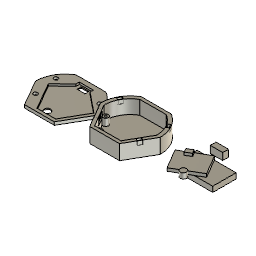
LampPost_Enclosure v37 (Autodesk Fusion 360 design; units mm, degrees)
Autodesk Fusion 360 part; units mm, degrees
note: some values were not read from the file. Set by a fixed rule: which sketch regions a step uses.
sketch "Sketch1" plane through (0, 0, 0) normal (0, 0, 1) x (1, 0, 0)
  line L0 (17.2286, 28.7143) -> (-16.253, 29.2775)
  line L1 (-33.4816, 0.5632) -> (-17.2286, -28.7143)
  line L2 (-17.2286, -28.7143) -> (16.253, -29.2775)
  line L3 (16.253, -29.2775) -> (33.4816, -0.5632)
  line L4 (19.6049, 32.6749) -> (-18.4948, 33.3158)
  line L5 (-38.0997, 0.6409) -> (-19.6049, -32.6749)
  line L6 (-19.6049, -32.6749) -> (18.4948, -33.3158)
  line L7 (18.4948, -33.3158) -> (38.0997, -0.6409)
  circle A0 centre (0, 0) radius 33.4863
  circle A1 centre (0, 0) radius 38.1051
  dimension "d1" = 29
  dimension "d2" = 33
  constraint coincident A0.centre A1.centre
  constraint coincident L3.end A0
  constraint coincident L7.end A1
  measures "d1" distance of A0.centre L3
  measures "d2" distance of A0.centre L7
extrude "Extrude1" add sketch "Sketch1" along normal blind 19 contours L0 L1 L2 L3 A0 | L4 L7 A0 A1 | L0 L4 A0 | L4 L5 A0 A1 | L1 L5 A0 | L3 L7 A0 | L5 L6 A0 | L2 L6 A0 | L6 L7 A0 makes body 1
sketch "Sketch2" plane through (0, 0, 19) normal (0, 0, 1) x (-1, 0, 0)
  arc A0 (-38.0997, 0.6409) -> (-19.6049, -32.6749) centre (0, 0) ccw
  line L0 (-19.6049, -32.6749) -> (18.4948, -33.3158)
  arc A1 (18.4948, -33.3158) -> (38.0997, -0.6409) centre (0, 0) ccw
  line L1 (38.0997, -0.6409) -> (19.6049, 32.6749)
  line L2 (19.6049, 32.6749) -> (-18.4948, 33.3158)
  line L3 (-18.4948, 33.3158) -> (-38.0997, 0.6409)
  line L4 (17.1219, 28.778) -> (-16.3615, 29.217)
  line L5 (-16.3615, 29.217) -> (-33.4834, 0.439)
  line L6 (-33.4834, 0.439) -> (-17.1219, -28.778)
  line L7 (-17.1219, -28.778) -> (16.3615, -29.217)
  line L8 (16.3615, -29.217) -> (33.4834, -0.439)
  line L9 (33.4834, -0.439) -> (17.1219, 28.778)
  line L10 (19.4836, 32.7474) -> (-18.6183, 33.2469)
  line L11 (-18.6183, 33.2469) -> (-38.1018, 0.4996)
  line L12 (-19.4836, -32.7474) -> (18.6183, -33.2469)
  line L13 (38.1018, -0.4996) -> (19.4836, 32.7474)
  circle A2 centre (0, 0) radius 33.4863
  dimension "d5" = 29
  dimension "d6" = 33
  constraint coincident A0.centre A1.centre
  constraint coincident L8.end A2
  measures "d5" distance of A0.centre L9
  measures "d6" distance of A0.centre L13
extrude "Extrude2" cut sketch "Sketch2" against normal blind 17.5 contours L4 L5 L6 L7 L8 L9 | L6 A2 | L8 A2 bodies 1
sketch "Sketch3" plane through (0, 0, 1.5) normal (0, 0, 1) x (-1, 0, 0)
  line L0 (33.4834, -0.439) -> (17.1219, 28.778)
  line L1 (17.1219, 28.778) -> (-16.3615, 29.217)
  line L2 (-16.3615, 29.217) -> (-33.4834, 0.439)
  arc A0 (-33.4834, 0.439) -> (-17.1219, -28.778) centre (0, 0) ccw
  line L3 (-17.1219, -28.778) -> (16.3615, -29.217)
  arc A1 (16.3615, -29.217) -> (33.4834, -0.439) centre (0, 0) ccw
  line L4 (133, 19.0526) -> (100, 38.1051)
  line L5 (67, 19.0526) -> (67, -19.0526)
  line L6 (67, -19.0526) -> (100, -38.1051)
  line L7 (100, -38.1051) -> (133, -19.0526)
  circle A2 centre (100, 0) radius 38.1051
  point P0 (100, 0)
  constraint coincident P0 A2.centre
  constraint coincident L4.start A2
extrude "Extrude3" add sketch "Sketch3" along normal blind 4 separate body contours L4 L5 L6 L7 A2 makes body 2
sketch "Sketch4" plane through (0, 0, 19) normal (0, 0, 1) x (-1, 0, 0)
  line L0 (-16.3615, 29.217) -> (17.1219, 28.778)
  line L1 (17.1219, 28.778) -> (33.4834, -0.439)
  arc A0 (16.3615, -29.217) -> (33.4834, -0.439) centre (0, 0) ccw
  line L2 (16.3615, -29.217) -> (-17.1219, -28.778)
  arc A1 (-33.4834, 0.439) -> (-17.1219, -28.778) centre (0, 0) ccw
  line L3 (-33.4834, 0.439) -> (-16.3615, 29.217)
  arc A2 (-38.0997, 0.6409) -> (-19.6049, -32.6749) centre (0, 0) ccw
  line L4 (-19.6049, -32.6749) -> (18.4948, -33.3158)
  arc A3 (18.4948, -33.3158) -> (38.0997, -0.6409) centre (0, 0) ccw
  line L5 (38.0997, -0.6409) -> (19.6049, 32.6749)
  line L6 (19.6049, 32.6749) -> (-18.4948, 33.3158)
  line L7 (-18.4948, 33.3158) -> (-38.0997, 0.6409)
  line L8 (-17.1219, -28.778) -> (-0.3802, -28.9975) construction
  line L9 (-0.3802, -28.9975) -> (-0.5551, -32.9953) construction
  line L10 (-17.1219, -28.778) -> (-17.155, -30.7472) construction
  line L11 (-17.155, -30.7472) -> (-0.4676, -30.9964) construction
  line L12 (-16.3615, 29.217) -> (0.3802, 28.9975) construction
  line L13 (0.3802, 28.9975) -> (0.5551, 32.9953) construction
  line L14 (17.1219, 28.778) -> (17.155, 30.7467) construction
  line L15 (17.155, 30.7467) -> (0.4676, 30.9964) construction
  line L16 (17.1219, 28.778) -> (25.3026, 14.1696) construction
  line L17 (25.3026, 14.1696) -> (28.8523, 16.017) construction
  line L18 (17.1219, 28.778) -> (18.8976, 29.7638)
  line L19 (18.8976, 29.7638) -> (27.0775, 15.0933) construction
  line L20 (-33.4834, 0.439) -> (-24.9226, 14.8279) construction
  line L21 (-24.9226, 14.8279) -> (-28.2973, 16.9784) construction
  line L22 (-33.4834, 0.439) -> (-35.225, 1.4839) construction
  line L23 (-35.225, 1.4839) -> (-26.6099, 15.9031) construction
  dimension "d12" = 1.9695
  dimension "d13" = 1.969
  dimension "d14" = 16.743
  dimension "d15" = 2.031
  dimension "d16" = 16.743
  dimension "d17" = 2.031
  constraint coincident L2.end A1.end
  constraint midpoint L2 L8.end
  constraint midpoint L4 L9.end
  constraint perpendicular L4 L10
  constraint midpoint L9 L11.end
  constraint coincident L0.start L3.end
  constraint midpoint L0 L12.end
  constraint midpoint L6 L13.end
  constraint coincident L0.end L1.start
  constraint perpendicular L6 L14
  constraint midpoint L13 L15.end
  constraint parallel L1 L16
  constraint midpoint L5 L17.end
  constraint perpendicular L5 L18
  constraint midpoint L17 L19.end
  constraint coincident A1.start L3.start
  constraint parallel L3 L20
  constraint midpoint L7 L21.end
  constraint perpendicular L7 L22
  constraint midpoint L21 L23.end
  measures "d12" distance of L2.end L10.end
  measures "d13" distance of L0.end L14.end
  measures "d14" distance of L0.end L16.end
  measures "d15" distance of L0.end L18.end
  measures "d16" distance of A1.start L20.end
  measures "d17" distance of A1.start L22.end
sketch "Sketch5" plane through (0, 0, 0) normal (0, 0, 1) x (1, 0, 0)
  line L0 (130, 0) -> (100, 0)
  line L1 (100, 0) -> (100, 50)
  line L2 (100, 50) -> (130, 50)
  line L3 (130, 50) -> (130, 0)
  dimension "d18" = 30
  dimension "d19" = 50
  constraint horizontal L0
  constraint vertical L1
  constraint horizontal L2
  constraint vertical L3
  measures "d18" distance of L0.start L0.end
  measures "d19" distance of L0.start L2.end
extrude "Extrude4" add sketch "Sketch5" along normal blind 7 separate body makes body 3
move_body "Move1" bodies 3 to x (0, 1, 0) y (-1, 0, 0) z (0, 0, 1) at (24.4081, -110.5598, 0)
move_body "Move2" bodies 3 to x (1, 0, 0) y (0, 1, 0) z (0, 0, 1) at (0, 0, 1.5)
sketch "Sketch6" plane through (0, 0, 19) normal (0, 0, 1) x (-1, 0, 0)
  line L0 (-100, 0) -> (-63, 0)
  line L1 (-63, 0) -> (-63, -29)
  line L2 (-63, -29) -> (-100, -29)
  line L3 (-100, -29) -> (-100, 0)
  line L4 (-100, 0) -> (-90, 0)
  line L5 (-90, 0) -> (-82, 0)
  line L6 (-82, 0) -> (-82, -6)
  line L7 (-82, -6) -> (-90, -6)
  line L8 (-90, -6) -> (-90, 0)
  dimension "d22" = 37
  dimension "d23" = 29
  dimension "d24" = 10
  dimension "d25" = 8
  dimension "d26" = 6
  constraint horizontal L0
  constraint vertical L1
  constraint horizontal L2
  constraint vertical L3
  constraint perpendicular L3 L4
  constraint horizontal L5
  constraint vertical L6
  constraint horizontal L7
  constraint vertical L8
  measures "d22" distance of L0.start L0.end
  measures "d23" distance of L0.start L2.end
  measures "d24" distance of L0.start L4.end
  measures "d25" distance of L4.end L5.end
  measures "d26" distance of L4.end L7.end
extrude "Extrude5" add sketch "Sketch6" along normal blind 4 separate body makes body 4
sketch "Sketch7" plane through (0, 0, 23) normal (0, 0, 1) x (-1, 0, 0)
  line L0 (-63, 0) -> (-100, 0)
  line L1 (-100, 0) -> (-100, -29)
  line L2 (-100, -29) -> (-63, -29)
  line L3 (-63, -29) -> (-63, 0)
  line L4 (-90, -1) -> (-82, -1)
  line L5 (-82, -1) -> (-82, -7)
  line L6 (-82, -7) -> (-90, -7)
  line L7 (-90, -7) -> (-90, -1)
  constraint horizontal L4
  constraint vertical L5
  constraint horizontal L6
  constraint vertical L7
move_body "Move3" bodies 4 to x (1, 0, 0) y (0, 1, 0) z (0, 0, 1) at (0, 0.8273, 0)
extrude "Extrude6" add sketch "Sketch7" along normal blind 3.5 contours L4 L5 L6 L7 bodies 4
move_body "Move4" bodies 4 to x (-0.017452, -0.999848, 0) y (0.999848, -0.017452, 0) z (0, 0, 1) at (-14.8475, 71.7391, 0)
move_body "Move5" bodies 4 to x (1, 0, 0) y (0, 1, 0) z (0, 0, 1) at (0.467, -0.1168, 0)
move_body "Move6" bodies 4 to x (1, 0, 0) y (0, 1, 0) z (0, 0, 1) at (0, 0, -7.5)
move_body "Move7" bodies 4 to x (1, 0, 0) y (0, 1, 0) z (0, 0, 1) at (0, 0, -5)
move_body "Move8" bodies 4 to x (1, 0, 0) y (0, 1, 0) z (0, 0, 1) at (0, 0, 5)
move_body "Move9" bodies 4 3 to x (1, 0, 0) y (0, 1, 0) z (0, 0, 1) at (95, 0, 0)
move_body "Move10" bodies 4 to x (1, 0, 0) y (0, 1, 0) z (0, 0, 1) at (0, 0, -3)
move_body "Move11" bodies 4 to x (1, 0, 0) y (0, 1, 0) z (0, 0, 1) at (0, 0, 0.5)
move_body "Move12" bodies 4 3 to x (1, 0, 0) y (0, 1, 0) z (0, 0, 1) at (-95, 0, 0)
sketch "Sketch8" plane through (0, 0, 0) normal (0, 0, 1) x (1, 0, 0)
  line L0 (0, 70) -> (-7.5, 70)
  line L1 (-7.5, 70) -> (-7.5, 86)
  line L2 (-7.5, 86) -> (0, 86)
  line L3 (0, 86) -> (0, 70)
  dimension "d31" = 7.5
  dimension "d32" = 16
  constraint horizontal L0
  constraint vertical L1
  constraint horizontal L2
  constraint vertical L3
  measures "d31" distance of L0.start L0.end
  measures "d32" distance of L0.start L2.end
extrude "Extrude7" add sketch "Sketch8" along normal blind 9 separate body makes body 5
move_body "Move13" bodies 5 to x (0, -1, 0) y (1, 0, 0) z (0, 0, 1) at (-78.7049, 19.5356, 12.5)
sketch "Sketch9" plane through (0, 0, 0) normal (0, 0, 1) x (1, 0, 0)
  circle A0 centre (0, -50) radius 4
  dimension "d35" = 8
  measures "d35" diameter of A0
extrude "Extrude8" add sketch "Sketch9" along normal blind 7 separate body makes body 6
move_body "Move14" bodies 6 to x (1, 0, 0) y (0, 1, 0) z (0, 0, 1) at (0, 52, 14)
move_body "Move15" bodies 6 3 4 to x (1, 0, 0) y (0, 1, 0) z (0, 0, 1) at (80, 0, 0)
move_body "Move16" bodies 6 to x (1, 0, 0) y (0, 1, 0) z (0, 0, 1) at (0, 0, -1)
move_body "Move17" bodies 6 4 3 to x (1, 0, 0) y (0, 1, 0) z (0, 0, 1) at (-80, 0, 0)
move_body "Move18" bodies 4 to x (0.5, -0.866025, 0) y (0.866025, 0.5, 0) z (0, 0, 1) at (17.3641, -27.6904, 0)
move_body "Move19" bodies 4 to x (1, 0, 0) y (0, 1, 0) z (0, 0, 1) at (-17.4314, 28.0362, 0)
move_body "Move20" bodies 3 to x (1, 0, 0) y (0, 1, 0) z (0, 0, 1) at (1.0034, -1.8395, 0)
move_body "Move21" bodies 6 to x (1, 0, 0) y (0, 1, 0) z (0, 0, 1) at (-0.2172, -24.4176, 0)
move_body "Move22" bodies 6 to x (1, 0, 0) y (0, 1, 0) z (0, 0, 1) at (0, 0, -1)
move_body "Move23" bodies 6 5 4 3 to x (1, 0, 0) y (0, 1, 0) z (0, 0, 1) at (110, 0, 0)
move_body "Move24" bodies 1 to x (0.999848, 0.017452, 0) y (-0.017452, 0.999848, 0) z (0, 0, 1) at (-0.5872, 0.6599, 0)
sketch "Sketch10" plane through (0, 0, 19) normal (0, 0, 1) x (-1, 0, 0)
  line L0 (-16.2817, 28.2672) -> (17.2043, 28.4126)
  line L1 (17.2043, 28.4126) -> (34.0732, -0.5144)
  arc A0 (17.4562, -29.5869) -> (34.0732, -0.5144) centre (0.5872, -0.6599) ccw
  line L2 (17.4562, -29.5869) -> (-16.0298, -29.7323)
  arc A1 (-32.8988, -0.8053) -> (-16.0298, -29.7323) centre (0.5872, -0.6599) ccw
  line L3 (-32.8988, -0.8053) -> (-16.2817, 28.2672)
  arc A2 (-37.5179, -0.684) -> (-18.4444, -33.6719) centre (0.5872, -0.6599) ccw
  line L4 (-18.4444, -33.6719) -> (19.6607, -33.6478)
  arc A3 (19.6607, -33.6478) -> (38.6924, -0.6358) centre (0.5872, -0.6599) ccw
  line L5 (38.6924, -0.6358) -> (19.6189, 32.3522)
  line L6 (19.6189, 32.3522) -> (-18.4862, 32.3281)
  line L7 (-18.4862, 32.3281) -> (-37.5179, -0.684)
  line L8 (17.4562, -29.5869) -> (0.7133, -29.6596) construction
  line L9 (17.4562, -29.5869) -> (17.4575, -31.6179) construction
  line L10 (17.4575, -31.6179) -> (0.7132, -31.6285) construction
  line L11 (0.7132, -31.6285) -> (0.7133, -29.6596) construction
  line L12 (0.7132, -31.6285) -> (0.7142, -33.2285)
  line L13 (0.7132, -31.6285) -> (0.7122, -30.0285)
  line L14 (0.7142, -33.2285) -> (-1.8858, -33.2301)
  line L15 (0.7122, -30.0285) -> (-1.8878, -30.0301)
  line L16 (-1.8878, -30.0301) -> (-1.8858, -33.2301)
  line L17 (0.7142, -33.2285) -> (3.3142, -33.2268)
  line L18 (0.7122, -30.0285) -> (3.3122, -30.0268)
  line L19 (3.3142, -33.2268) -> (3.3122, -30.0268)
  line L20 (-16.2817, 28.2672) -> (-24.5901, 13.7311) construction
  line L21 (-24.5901, 13.7311) -> (-26.2996, 14.7082) construction
  line L22 (-26.2996, 14.7082) -> (-27.6858, 15.5073)
  line L23 (-26.2996, 14.7082) -> (-24.9105, 13.9142)
  line L24 (-27.6858, 15.5073) -> (-26.3872, 17.7598)
  line L25 (-24.9105, 13.9142) -> (-23.6203, 16.1715)
  line L26 (-27.6858, 15.5073) -> (-28.9843, 13.2548)
  line L27 (-24.9105, 13.9142) -> (-26.2007, 11.6569)
  line L28 (-26.2007, 11.6569) -> (-28.9843, 13.2548)
  line L29 (-23.6203, 16.1715) -> (-26.3872, 17.7598)
  line L30 (34.0732, -0.5144) -> (25.6389, 13.9489) construction
  line L31 (25.6389, 13.9489) -> (27.3703, 14.95) construction
  line L32 (27.3703, 14.95) -> (28.7554, 15.7509)
  line L33 (27.3703, 14.95) -> (25.9851, 14.1492)
  line L34 (25.9851, 14.1492) -> (27.2866, 11.8983)
  line L35 (28.7554, 15.7509) -> (30.0568, 13.5001)
  line L36 (28.7554, 15.7509) -> (27.454, 18.0018)
  line L37 (25.9851, 14.1492) -> (24.6837, 16.4)
  line L38 (30.0568, 13.5001) -> (27.2866, 11.8983)
  line L39 (27.454, 18.0018) -> (24.6837, 16.4)
  line L40 (17.2043, 28.4126) -> (0.4615, 28.3399) construction
  line L41 (0.4615, 28.3399) -> (0.4602, 30.3399) construction
  line L42 (0.4602, 30.3399) -> (0.4612, 28.7399)
  line L43 (0.4602, 30.3399) -> (0.4532, 31.9399)
  line L44 (0.4612, 28.7399) -> (-2.1388, 28.7382)
  line L45 (0.4532, 31.9399) -> (-2.1467, 31.9286)
  line L46 (0.4612, 28.7399) -> (3.0612, 28.7415)
  line L47 (0.4532, 31.9399) -> (3.0532, 31.9511)
  line L48 (3.0612, 28.7415) -> (3.0532, 31.9511)
  line L49 (-2.1388, 28.7382) -> (-2.1467, 31.9286)
  dimension "d38" = 16.743
  dimension "d39" = 2.031
  dimension "d40" = 1.6
  dimension "d41" = 1.6
  dimension "d42" = 2.6
  dimension "d43" = 2.6
  dimension "d44" = 2.6
  dimension "d45" = 2.6
  dimension "d46" = 16.743
  dimension "d48" = 1.969
  dimension "d49" = 1.6
  dimension "d50" = 1.6
  dimension "d51" = 2.6
  dimension "d52" = 2.6
  dimension "d53" = 2.6
  dimension "d54" = 2.6
  dimension "d55" = 16.743
  dimension "d56" = 2
  dimension "d57" = 1.6
  dimension "d58" = 1.6
  dimension "d59" = 2.6
  dimension "d60" = 2.6
  dimension "d61" = 2.6
  dimension "d62" = 2.6
  dimension "d63" = 16.743
  dimension "d64" = 2
  dimension "d65" = 1.6
  dimension "d66" = 1.6
  dimension "d67" = 2.6
  dimension "d68" = 2.6
  dimension "d69" = 2.6
  dimension "d70" = 2.6
  constraint coincident A0.start L2.start
  constraint parallel L2 L8
  constraint perpendicular L4 L9
  constraint perpendicular L9 L10
  constraint perpendicular L10 L12
  constraint perpendicular L10 L13
  constraint perpendicular L12 L14
  constraint perpendicular L13 L15
  constraint perpendicular L12 L17
  constraint perpendicular L13 L18
  constraint coincident L0.start L3.end
  constraint parallel L3 L20
  constraint perpendicular L3 L21
  constraint perpendicular L7 L22
  constraint parallel L21 L23
  constraint perpendicular L22 L24
  constraint perpendicular L23 L25
  constraint perpendicular L22 L26
  constraint perpendicular L21 L27
  constraint coincident L1.end A0.end
  constraint parallel L1 L30
  constraint perpendicular L5 L31
  constraint parallel L31 L32
  constraint parallel L31 L33
  constraint perpendicular L31 L34
  constraint perpendicular L32 L35
  constraint perpendicular L32 L36
  constraint perpendicular L31 L37
  constraint coincident L0.end L1.start
  constraint parallel L0 L40
  constraint perpendicular L6 L41
  constraint parallel L41 L42
  constraint perpendicular L0 L43
  constraint perpendicular L42 L44
  constraint perpendicular L43 L45
  constraint perpendicular L41 L46
  constraint perpendicular L43 L47
  measures "d38" distance of A0.start L8.end
  measures "d39" distance of A0.start L9.end
  measures "d40" distance of L10.end L12.end
  measures "d41" distance of L10.end L13.end
  measures "d42" distance of L12.end L14.end
  measures "d43" distance of L13.end L15.end
  measures "d44" distance of L12.end L17.end
  measures "d45" distance of L13.end L18.end
  measures "d46" distance of L0.start L20.end
  measures "d48" distance of L20.end L21.end
  measures "d49" distance of L21.end L22.end
  measures "d50" distance of L21.end L23.end
  measures "d51" distance of L22.end L24.end
  measures "d52" distance of L23.end L25.end
  measures "d53" distance of L22.end L26.end
  measures "d54" distance of L23.end L27.end
  measures "d55" distance of L1.end L30.end
  measures "d56" distance of L30.end L31.end
  measures "d57" distance of L31.end L32.end
  measures "d58" distance of L31.end L33.end
  measures "d59" distance of L33.end L34.end
  measures "d60" distance of L32.end L35.end
  measures "d61" distance of L32.end L36.end
  measures "d62" distance of L33.end L37.end
  measures "d63" distance of L0.end L40.end
  measures "d64" distance of L40.end L41.end
  measures "d65" distance of L41.end L42.end
  measures "d66" distance of L41.end L43.end
  measures "d67" distance of L42.end L44.end
  measures "d68" distance of L43.end L45.end
  measures "d69" distance of L42.end L46.end
  measures "d70" distance of L43.end L47.end
extrude "Extrude9" cut sketch "Sketch10" against normal blind 5.1 contours L12 L13 L17 L18 L19 | L12 L13 L14 L15 L16 bodies 1
extrude "Extrude10" cut sketch "Sketch10" against normal blind 5.1 contours L22 L23 L26 L27 L28 | L22 L23 L24 L25 L29 bodies 1
extrude "Extrude11" cut sketch "Sketch10" against normal blind 5.1 contours L42 L43 L46 L47 L48 | L42 L43 L44 L45 L49 bodies 1
move_body "Move25" bodies 2 to x (-0.866025, -0.5, 0) y (0.5, -0.866025, 0) z (0, 0, 1) at (-238.6551, -140.1577, 0)
move_body "Move26" bodies 2 to x (1, 0, 0) y (0, 1, 0) z (0, 0, 1) at (67.9441, 89.5203, 0)
sketch "Sketch11" plane through (0, 0, 5.5) normal (0, 0, 1) x (-1, 0, 0)
  arc A0 (46.0033, 0.6373) -> (65.0559, -32.3627) centre (84.1085, 0.6373) ccw
  line L0 (65.0559, -32.3627) -> (103.161, -32.3627)
  arc A1 (103.161, -32.3627) -> (122.2136, 0.6373) centre (84.1085, 0.6373) ccw
  line L1 (122.2136, 0.6373) -> (103.161, 33.6373)
  line L2 (103.161, 33.6373) -> (65.0559, 33.6373)
  line L3 (65.0559, 33.6373) -> (46.0033, 0.6373)
  line L4 (103.161, -32.3627) -> (65.0559, -32.3627) construction
  line L5 (65.0559, -32.3627) -> (65.0559, -28.3627) construction
  line L6 (65.0559, -28.3627) -> (103.161, -28.3627) construction
  line L7 (103.161, -28.3627) -> (103.161, -32.3627) construction
  line L8 (103.161, -28.3627) -> (84.1085, -28.3627) construction
  line L9 (84.1085, -28.3627) -> (84.1085, -26.3627) construction
  line L10 (84.1085, -26.3627) -> (75.1085, -26.3627)
  line L11 (84.1085, -26.3627) -> (93.1085, -26.3627)
  line L12 (75.1085, -26.3627) -> (75.1085, -17.8627)
  line L13 (93.1085, -26.3627) -> (93.1085, -17.8627)
  line L14 (93.1085, -17.8627) -> (75.1085, -17.8627)
  line L15 (84.1085, -26.3627) -> (84.1085, -22.1127) construction
  line L16 (84.1085, -22.1127) -> (84.1085, -19.6127)
  line L17 (84.1085, -22.1127) -> (84.1085, -24.6127)
  line L18 (84.1085, -24.6127) -> (79.1085, -24.6127)
  line L19 (84.1085, -19.6127) -> (79.1085, -19.6127)
  line L20 (84.1085, -24.6127) -> (89.1085, -24.6127)
  line L21 (84.1085, -19.6127) -> (89.1085, -19.6127)
  line L22 (89.1085, -24.6127) -> (89.1085, -19.6127)
  line L23 (79.1085, -24.6127) -> (79.1085, -19.6127)
  line L24 (103.161, 33.6373) -> (65.0559, 33.6373) construction
  line L25 (65.0559, 33.6373) -> (65.0559, 29.6373) construction
  line L26 (65.0559, 29.6373) -> (103.161, 29.6373) construction
  line L27 (103.161, 29.6373) -> (103.161, 33.6373) construction
  line L28 (103.161, 33.6373) -> (84.1085, 33.6373) construction
  line L29 (84.1085, 33.6373) -> (84.1085, 23.5123) construction
  circle A2 centre (84.1085, 23.5123) radius 4.125
  dimension "d77" = 4
  dimension "d78" = 2
  dimension "d79" = 9
  dimension "d80" = 9
  dimension "d81" = 8.5
  dimension "d82" = 8.5
  dimension "d83" = 4.25
  dimension "d84" = 2.5
  dimension "d85" = 2.5
  dimension "d86" = 5
  dimension "d87" = 5
  dimension "d88" = 5
  dimension "d89" = 5
  dimension "d90" = 4
  dimension "d91" = 19.0525
  dimension "d92" = 10.125
  dimension "d93" = 8.25
  constraint horizontal L4
  constraint vertical L5
  constraint horizontal L6
  constraint vertical L7
  constraint coincident L0.end A1.start
  constraint midpoint L6 L8.end
  constraint perpendicular L6 L9
  constraint perpendicular L9 L10
  constraint perpendicular L9 L11
  constraint perpendicular L10 L12
  constraint perpendicular L11 L13
  constraint perpendicular L14 L15
  constraint parallel L15 L16
  constraint perpendicular L11 L17
  constraint perpendicular L15 L18
  constraint perpendicular L16 L19
  constraint perpendicular L15 L20
  constraint perpendicular L16 L21
  constraint horizontal L24
  constraint vertical L25
  constraint horizontal L26
  constraint vertical L27
  constraint coincident L1.end L2.start
  constraint perpendicular L25 L28
  constraint perpendicular L26 L29
  constraint coincident L29.end A2.centre
  measures "d77" distance of L0.end L6.end
  measures "d78" distance of L8.end L9.end
  measures "d79" distance of L9.end L10.end
  measures "d80" distance of L9.end L11.end
  measures "d81" distance of L10.end L12.end
  measures "d82" distance of L11.end L13.end
  measures "d83" distance of L9.end L15.end
  measures "d84" distance of L15.end L16.end
  measures "d85" distance of L15.end L17.end
  measures "d86" distance of L17.end L18.end
  measures "d87" distance of L16.end L19.end
  measures "d88" distance of L17.end L20.end
  measures "d89" distance of L16.end L21.end
  measures "d90" distance of L1.end L26.end
  measures "d91" distance of L1.end L28.end
  measures "d92" distance of L28.end L29.end
  measures "d93" diameter of A2
move_body "Move27" bodies 6 5 4 3 to x (1, 0, 0) y (0, 1, 0) z (0, 0, 1) at (-274.039, -1.8555, 0)
extrude "Extrude12" cut sketch "Sketch11" against normal blind 10 contours L16 L17 L18 L19 L23 | L16 L17 L20 L21 L22 bodies 2
extrude "Extrude13" cut sketch "Sketch11" against normal blind 2.5 contours L10 L11 L12 L13 L14 bodies 2
extrude "Extrude14" cut sketch "Sketch11" against normal blind 10 contours A2 bodies 2
sketch "Sketch12" plane through (0, 0, 5.5) normal (0, 0, 1) x (-1, 0, 0)
  circle A0 centre (84.1085, 23.5123) radius 4.125
  line L0 (93.1085, -17.8627) -> (93.1085, -26.3627)
  line L1 (93.1085, -26.3627) -> (75.1085, -26.3627)
  line L2 (75.1085, -26.3627) -> (75.1085, -17.8627)
  line L3 (75.1085, -17.8627) -> (93.1085, -17.8627)
  arc A1 (46.0033, 0.6373) -> (65.0559, -32.3627) centre (84.1085, 0.6373) ccw
  line L4 (65.0559, -32.3627) -> (103.161, -32.3627)
  arc A2 (103.161, -32.3627) -> (122.2136, 0.6373) centre (84.1085, 0.6373) ccw
  line L5 (122.2136, 0.6373) -> (103.161, 33.6373)
  line L6 (103.161, 33.6373) -> (65.0559, 33.6373)
  line L7 (65.0559, 33.6373) -> (46.0033, 0.6373)
  line L8 (122.2136, 0.6373) -> (112.6873, 17.1373) construction
  line L9 (112.6873, 17.1373) -> (110.9553, 16.1373) construction
  line L10 (110.9553, 16.1373) -> (109.5696, 15.3373) construction
  line L11 (110.9553, 16.1373) -> (112.3409, 16.9373) construction
  line L12 (109.5696, 15.3373) -> (108.2696, 17.589) construction
  line L13 (109.5696, 15.3373) -> (110.8696, 13.0856) construction
  line L14 (112.3409, 16.9373) -> (113.6409, 14.6856) construction
  line L15 (112.3409, 16.9373) -> (111.0409, 19.189) construction
  line L16 (113.6409, 14.6856) -> (110.8696, 13.0856) construction
  line L17 (108.2696, 17.589) -> (111.0409, 19.189) construction
  line L18 (109.5696, 15.3373) -> (110.4357, 15.8373)
  line L19 (109.5696, 15.3373) -> (105.9323, 13.2373)
  circle A3 centre (108.184, 14.5373) radius 2.6
  dimension "d100" = 19.0525
  dimension "d101" = 2
  dimension "d102" = 1.6
  dimension "d103" = 1.6
  dimension "d104" = 2.6
  dimension "d105" = 2.6
  dimension "d106" = 2.6
  dimension "d107" = 2.6
  dimension "d108" = 1
  dimension "d109" = 4.2
  constraint coincident A2.end L5.start
  constraint parallel L5 L8
  constraint perpendicular L5 L9
  constraint perpendicular L5 L10
  constraint perpendicular L5 L11
  constraint perpendicular L10 L12
  constraint perpendicular L10 L13
  constraint perpendicular L9 L14
  constraint perpendicular L9 L15
  constraint perpendicular L13 L18
  constraint perpendicular L13 L19
  constraint coincident L19.end A3
  constraint coincident L18.end A3
  measures "d100" distance of A2.end L8.end
  measures "d101" distance of L8.end L9.end
  measures "d102" distance of L9.end L10.end
  measures "d103" distance of L9.end L11.end
  measures "d104" distance of L10.end L12.end
  measures "d105" distance of L10.end L13.end
  measures "d106" distance of L11.end L14.end
  measures "d107" distance of L11.end L15.end
  measures "d108" distance of L10.end L18.end
  measures "d109" distance of L10.end L19.end
extrude "Extrude15" cut sketch "Sketch12" against normal blind 3.1 contours L18 L19 A3 | L18 L19 A3 bodies 2
extrude "Extrude16" add 1 faces at (-1.5795, 31.0946, 13.9) along direction (0, 0, 1) blind 5.1 on bodies 1 bodies 1
extrude "Extrude17" add 1 faces at (-1.3226, -30.8737, 13.9) along direction (0, 0, 1) blind 5.1 on bodies 1 bodies 1
sketch "Sketch13" plane through (0, 0, 19) normal (0, 0, 1) x (-1, 0, 0)
  line L0 (-26.3872, 17.7598) -> (-23.6203, 16.1715)
  line L1 (-23.6203, 16.1715) -> (-26.2007, 11.6569)
  line L2 (-26.2007, 11.6569) -> (-28.9843, 13.2548)
  line L3 (-28.9843, 13.2548) -> (-26.3872, 17.7598)
  line L4 (-16.2817, 28.2672) -> (17.2043, 28.4126)
  line L5 (17.2043, 28.4126) -> (34.0732, -0.5144)
  arc A0 (17.4562, -29.5869) -> (34.0732, -0.5144) centre (0.5872, -0.6599) ccw
  line L6 (17.4562, -29.5869) -> (-16.0298, -29.7323)
  arc A1 (-32.8988, -0.8053) -> (-16.0298, -29.7323) centre (0.5872, -0.6599) ccw
  line L7 (-32.8988, -0.8053) -> (-16.2817, 28.2672)
  arc A2 (-37.5179, -0.684) -> (-18.4444, -33.6719) centre (0.5872, -0.6599) ccw
  line L8 (-18.4444, -33.6719) -> (19.6607, -33.6478)
  arc A3 (19.6607, -33.6478) -> (38.6924, -0.6358) centre (0.5872, -0.6599) ccw
  line L9 (38.6924, -0.6358) -> (19.6189, 32.3522)
  line L10 (19.6189, 32.3522) -> (-18.4862, 32.3281)
  line L11 (-18.4862, 32.3281) -> (-37.5179, -0.684)
  line L12 (-16.0298, -29.7323) -> (-24.4519, -15.2617) construction
  line L13 (-24.4519, -15.2617) -> (-30.0576, -18.5243) construction
  line L14 (-24.4519, -15.2617) -> (-17.9782, -15.2617) construction
  line L15 (-30.0576, -18.5243) -> (-31.4404, -19.3292)
  line L16 (-30.0576, -18.5243) -> (-28.6747, -17.7195)
  line L17 (-31.4404, -19.3292) -> (-32.7483, -17.082)
  line L18 (-31.4404, -19.3292) -> (-30.1326, -21.5763)
  line L19 (-28.6747, -17.7195) -> (-27.3669, -19.9666)
  line L20 (-28.6747, -17.7195) -> (-29.9826, -15.4724)
  line L21 (-27.3669, -19.9666) -> (-30.1326, -21.5763)
  line L22 (-29.9826, -15.4724) -> (-32.7483, -17.082)
  line L23 (17.4562, -29.5869) -> (25.777, -15.0579) construction
  line L24 (25.777, -15.0579) -> (31.4053, -18.2812) construction
  line L25 (25.777, -15.0579) -> (32.2506, -15.0579) construction
  line L26 (31.4053, -18.2812) -> (32.7938, -19.0764)
  line L27 (31.4053, -18.2812) -> (30.0169, -17.4861)
  line L28 (32.7938, -19.0764) -> (31.5016, -21.3326)
  line L29 (30.0169, -17.4861) -> (28.7248, -19.7423)
  line L30 (30.0169, -17.4861) -> (31.3091, -15.2299)
  line L31 (32.7938, -19.0764) -> (34.0859, -16.8202)
  line L32 (31.3091, -15.2299) -> (34.0859, -16.8202)
  line L33 (31.5016, -21.3326) -> (28.7248, -19.7423)
  dimension "d116" = 16.743
  dimension "d117" = 149.8
  dimension "d118" = 6.486
  dimension "d119" = 1.6
  dimension "d120" = 1.6
  dimension "d121" = 2.6
  dimension "d122" = 2.6
  dimension "d123" = 2.6
  dimension "d124" = 2.6
  dimension "d125" = 16.743
  dimension "d126" = 29.8
  dimension "d127" = 6.486
  dimension "d128" = 1.6
  dimension "d129" = 1.6
  dimension "d130" = 2.6
  dimension "d131" = 2.6
  dimension "d132" = 2.6
  dimension "d133" = 2.6
  constraint coincident L6.end A1.end
  constraint horizontal L14
  constraint perpendicular L12 L13
  constraint parallel L13 L15
  constraint parallel L13 L16
  constraint perpendicular L15 L17
  constraint perpendicular L15 L18
  constraint perpendicular L13 L19
  constraint perpendicular L13 L20
  constraint coincident A0.start L6.start
  constraint horizontal L25
  constraint perpendicular L23 L24
  constraint parallel L24 L26
  constraint parallel L24 L27
  constraint perpendicular L26 L28
  constraint perpendicular L24 L29
  constraint perpendicular L24 L30
  constraint perpendicular L26 L31
  measures "d116" distance of L6.end L12.end
  measures "d117" angle of L13 L14
  measures "d118" distance of L12.end L13.end
  measures "d119" distance of L13.end L15.end
  measures "d120" distance of L13.end L16.end
  measures "d121" distance of L15.end L17.end
  measures "d122" distance of L15.end L18.end
  measures "d123" distance of L16.end L19.end
  measures "d124" distance of L16.end L20.end
  measures "d125" distance of A0.start L23.end
  measures "d126" angle of L24 L25
  measures "d127" distance of L23.end L24.end
  measures "d128" distance of L24.end L26.end
  measures "d129" distance of L24.end L27.end
  measures "d130" distance of L26.end L28.end
  measures "d131" distance of L27.end L29.end
  measures "d132" distance of L27.end L30.end
  measures "d133" distance of L26.end L31.end
extrude "Extrude18" cut sketch "Sketch13" against normal blind 5.1 contours L15 L16 L18 L19 L21 | L15 L16 L17 L20 L22 bodies 1
extrude "Extrude19" cut sketch "Sketch13" against normal blind 5.1 contours L26 L27 L30 L31 L32 | L26 L27 L28 L29 L33 bodies 1
sketch "Sketch14" plane through (0, 0, 5.5) normal (0, 0, 1) x (-1, 0, 0)
  circle A0 centre (108.184, 14.5373) radius 2.6
  circle A1 centre (84.1085, 23.5123) radius 4.125
  line L0 (93.1085, -17.8627) -> (93.1085, -26.3627)
  line L1 (93.1085, -26.3627) -> (75.1085, -26.3627)
  line L2 (75.1085, -26.3627) -> (75.1085, -17.8627)
  line L3 (75.1085, -17.8627) -> (93.1085, -17.8627)
  arc A2 (46.0033, 0.6373) -> (65.0559, -32.3627) centre (84.1085, 0.6373) ccw
  line L4 (65.0559, -32.3627) -> (103.161, -32.3627)
  arc A3 (103.161, -32.3627) -> (122.2136, 0.6373) centre (84.1085, 0.6373) ccw
  line L5 (122.2136, 0.6373) -> (103.161, 33.6373)
  line L6 (103.161, 33.6373) -> (65.0559, 33.6373)
  line L7 (65.0559, 33.6373) -> (46.0033, 0.6373)
  line L8 (65.0559, -32.3627) -> (55.5297, -15.8627) construction
  line L9 (51.1085, -18.4152) -> (51.9745, -17.9152) construction
  line L10 (51.9745, -17.9152) -> (54.745, -16.3139) construction
  line L11 (54.745, -16.3139) -> (56.0461, -18.565) construction
  line L12 (51.9745, -17.9152) -> (53.2745, -20.1669) construction
  line L13 (56.0461, -18.565) -> (53.2745, -20.1669) construction
  line L14 (54.745, -16.3139) -> (53.444, -14.0629) construction
  line L15 (51.9745, -17.9152) -> (50.6745, -15.6636) construction
  line L16 (53.444, -14.0629) -> (50.6745, -15.6636) construction
  line L17 (54.745, -16.3139) -> (53.8792, -16.8143)
  line L18 (54.745, -16.3139) -> (58.3823, -14.2139)
  circle A4 centre (56.1308, -15.5141) radius 2.6
  line L19 (103.161, -32.3627) -> (112.6873, -15.8627) construction
  line L20 (112.6873, -15.8627) -> (117.1085, -18.4152) construction
  line L21 (117.1085, -18.4152) -> (116.2424, -17.9152) construction
  line L22 (116.2424, -17.9152) -> (113.4711, -16.3153) construction
  line L23 (113.4711, -16.3153) -> (114.7711, -14.0636) construction
  line L24 (116.2424, -17.9152) -> (117.5424, -15.6635) construction
  line L25 (113.4711, -16.3153) -> (112.1712, -18.5669) construction
  line L26 (116.2424, -17.9152) -> (114.9424, -20.1669) construction
  line L27 (112.1712, -18.5669) -> (114.9424, -20.1669) construction
  line L28 (117.5424, -15.6635) -> (114.7711, -14.0636) construction
  line L29 (113.4711, -16.3153) -> (114.3372, -16.8152)
  line L30 (113.4711, -16.3153) -> (109.8338, -14.2153)
  circle A5 centre (112.0855, -15.5153) radius 2.6
  dimension "d138" = 19.0525
  dimension "d139" = 1
  dimension "d140" = 3.2
  dimension "d141" = 2.6
  dimension "d142" = 2.6
  dimension "d143" = 2.6
  dimension "d144" = 2.6
  dimension "d145" = 1
  dimension "d146" = 4.2
  dimension "d147" = 19.0525
  dimension "d148" = 1
  dimension "d149" = 3.2
  dimension "d150" = 2.6
  dimension "d151" = 2.6
  dimension "d152" = 2.6
  dimension "d153" = 2.6
  dimension "d154" = 1
  dimension "d155" = 4.2
  constraint coincident A2.end L4.start
  constraint midpoint A2 L9.start
  constraint perpendicular L8 L9
  constraint perpendicular L10 L11
  constraint perpendicular L9 L12
  constraint perpendicular L10 L14
  constraint perpendicular L9 L15
  constraint coincident L10 L17.end
  constraint perpendicular L8 L18
  constraint coincident L17.end A4
  constraint coincident L18.end A4
  constraint coincident L4.end A3.start
  constraint midpoint A3 L20.end
  constraint perpendicular L19 L21
  constraint parallel L20 L22
  constraint perpendicular L20 L23
  constraint perpendicular L20 L24
  constraint perpendicular L22 L25
  constraint perpendicular L21 L26
  constraint perpendicular L23 L29
  constraint perpendicular L25 L30
  constraint coincident L30.end A5
  constraint coincident L29.end A5
  measures "d138" distance of A2.end L8.end
  measures "d139" distance of L9.start L9.end
  measures "d140" distance of L9.end L10.end
  measures "d141" distance of L10.end L11.end
  measures "d142" distance of L9.end L12.end
  measures "d143" distance of L10.end L14.end
  measures "d144" distance of L9.end L15.end
  measures "d145" distance of L10.end L17.end
  measures "d146" distance of L10.end L18.end
  measures "d147" distance of L4.end L19.end
  measures "d148" distance of L20.end L21.end
  measures "d149" distance of L21.end L22.end
  measures "d150" distance of L22.end L23.end
  measures "d151" distance of L21.end L24.end
  measures "d152" distance of L22.end L25.end
  measures "d153" distance of L21.end L26.end
  measures "d154" distance of L22.end L29.end
  measures "d155" distance of L22.end L30.end
extrude "Extrude20" cut sketch "Sketch14" against normal blind 3.1 contours L17 L18 A4 | L17 L18 A4 | L29 L30 A5 | L29 L30 A5 bodies 2
sketch "Sketch15" plane through (0, 0, 1.5) normal (0, 0, 1) x (-1, 0, 0)
  line L0 (34.0732, -0.5144) -> (17.2043, 28.4126)
  line L1 (17.2043, 28.4126) -> (-16.2817, 28.2672)
  line L2 (-16.2817, 28.2672) -> (-32.8988, -0.8053)
  arc A0 (-32.8988, -0.8053) -> (-16.0298, -29.7323) centre (0.5872, -0.6599) ccw
  line L3 (-16.0298, -29.7323) -> (17.4562, -29.5869)
  arc A1 (17.4562, -29.5869) -> (34.0732, -0.5144) centre (0.5872, -0.6599) ccw
  line L4 (34.0732, -0.5144) -> (31.6545, -1.925) construction
  line L5 (31.6545, -1.925) -> (29.2364, 2.2215) construction
  line L6 (29.2364, 2.2215) -> (17.9019, 21.658) construction
  circle A2 centre (17.9019, 21.658) radius 3.5
  circle A3 centre (29.2364, 2.2215) radius 3.5
  dimension "d158" = 2.8
  dimension "d159" = 4.8
  dimension "d160" = 22.5
  dimension "d161" = 7
  dimension "d162" = 7
  constraint coincident L0.start A1.end
  constraint perpendicular L0 L4
  constraint perpendicular L4 L5
  constraint perpendicular L4 L6
  constraint coincident L6.end A2.centre
  constraint coincident L5.end L6.start
  measures "d158" distance of L0.start L4.end
  measures "d159" distance of L4.end L5.end
  measures "d160" distance of L5.end L6.end
  measures "d161" diameter of A2
  measures "d162" diameter of A3
extrude "Extrude21" add sketch "Sketch15" along normal blind 9 contours L0 A3 picked at (29.4941, 1.1088) bodies 1
extrude "Extrude22" add sketch "Sketch15" along normal blind 9 contours L0 A2 picked at (18.7758, 20.7595) bodies 1
sketch "Sketch16" plane through (0, 0, 10.5) normal (0, 0, 1) x (-1, 0, 0)
  line L0 (32.7131, 1.818) -> (30.5973, 5.4461)
  arc A0 (30.5973, 5.4461) -> (32.7131, 1.818) centre (29.2364, 2.2215) ccw
  circle A1 centre (29.2364, 2.2215) radius 1.4
  dimension "d167" = 2.8
  constraint concentric A0 A1
  measures "d167" diameter of A1
sketch "Sketch17" plane through (0, 0, 10.5) normal (0, 0, 1) x (-1, 0, 0)
  line L0 (21.3786, 21.2545) -> (19.2628, 24.8826)
  arc A0 (19.2628, 24.8826) -> (21.3786, 21.2545) centre (17.9019, 21.658) ccw
  circle A1 centre (17.9019, 21.658) radius 1.4
  dimension "d168" = 2.8
  constraint concentric A0 A1
  measures "d168" diameter of A1
extrude "Extrude23" cut sketch "Sketch16" against normal blind 5 contours A1 bodies 1
extrude "Extrude24" cut sketch "Sketch17" against normal blind 5 contours A1 bodies 1
sketch "Sketch18" plane through (-25.2026, -14.697, 0) normal (0.863846, 0.503756, 0) x (-0.503756, 0.863846, 0)
  line L0 (-11.791, 1.5) -> (-11.791, 10.5)
  line L1 (-11.791, 10.5) -> (-7.591, 10.5)
  line L2 (-7.591, 10.5) -> (-7.591, 1.5)
  line L3 (-7.591, 1.5) -> (10.709, 1.5)
  line L4 (10.709, 1.5) -> (10.709, 10.5)
  line L5 (10.709, 10.5) -> (14.909, 10.5)
  line L6 (14.909, 10.5) -> (14.909, 1.5)
  line L7 (14.909, 1.5) -> (17.609, 1.5)
  line L8 (17.609, 1.5) -> (17.609, 19)
  line L9 (17.609, 19) -> (-15.8773, 19)
  line L10 (-15.8773, 19) -> (-15.8773, 1.5)
  line L11 (-15.8773, 1.5) -> (-11.791, 1.5)
  line L12 (17.609, 1.5) -> (4.809, 1.5) construction
  line L13 (4.809, 1.5) -> (4.809, 10.5) construction
  line L14 (4.809, 10.5) -> (4.809, 13) construction
  line L15 (4.809, 13) -> (4.809, 9)
  line L16 (4.809, 13) -> (4.809, 17)
  line L17 (4.809, 17) -> (10.809, 17)
  line L18 (4.809, 9) -> (10.809, 9)
  line L19 (10.809, 17) -> (10.809, 9)
  line L20 (4.809, 17) -> (-1.191, 17)
  line L21 (4.809, 9) -> (-1.191, 9)
  line L22 (-1.191, 17) -> (-1.191, 9)
  dimension "d173" = 12.8
  dimension "d174" = 9
  dimension "d175" = 2.5
  dimension "d176" = 4
  dimension "d177" = 4
  dimension "d178" = 6
  dimension "d179" = 6
  dimension "d180" = 6
  dimension "d181" = 6
  constraint coincident L7.end L8.start
  constraint perpendicular L8 L12
  constraint perpendicular L3 L13
  constraint parallel L13 L14
  constraint parallel L13 L15
  constraint parallel L14 L16
  constraint perpendicular L16 L17
  constraint perpendicular L15 L18
  constraint perpendicular L16 L20
  constraint perpendicular L15 L21
  measures "d173" distance of L7.end L12.end
  measures "d174" distance of L12.end L13.end
  measures "d175" distance of L13.end L14.end
  measures "d176" distance of L14.end L15.end
  measures "d177" distance of L14.end L16.end
  measures "d178" distance of L16.end L17.end
  measures "d179" distance of L15.end L18.end
  measures "d180" distance of L16.end L20.end
  measures "d181" distance of L15.end L21.end
extrude "Extrude25" cut sketch "Sketch18" against normal blind 11 contours L4 L5 L15 L16 L17 L18 L19 | L15 L16 L20 L21 L22 bodies 1
sketch "Sketch19" plane through (-28.7226, -16.6072, 0) normal (-0.865709, -0.500548, 0) x (0.500548, -0.865709, 0)
  line L0 (1.3141, 17) -> (1.3141, 9)
  line L1 (1.3141, 9) -> (-10.586, 9)
  line L2 (-10.586, 9) -> (-10.586, 10.5)
  line L3 (-10.586, 10.5) -> (-10.686, 10.5)
  line L4 (-10.686, 10.5) -> (-10.686, 17)
  line L5 (-10.686, 17) -> (1.3141, 17)
  line L6 (-19.9177, 0) -> (18.1874, 0)
  line L7 (18.1874, 0) -> (18.1874, 19)
  line L8 (18.1874, 19) -> (-19.9177, 19)
  line L9 (-19.9177, 19) -> (-19.9177, 0)
  line L10 (1.3141, 18) -> (-10.6676, 18)
  line L11 (-11.686, 17) -> (-11.686, 18)
  line L12 (-11.686, 18) -> (-10.6676, 18)
  line L13 (-11.686, 17) -> (-11.686, 9)
  line L14 (1.3141, 18) -> (2.3141, 18)
  line L15 (2.3141, 18) -> (2.3141, 9)
  line L16 (2.3141, 9) -> (2.3141, 8)
  line L17 (2.3141, 8) -> (-10.586, 8)
  line L18 (-11.686, 9) -> (-11.686, 8)
  line L19 (-11.686, 8) -> (-10.586, 8)
  dimension "d184" = 1
  dimension "d185" = 1
  dimension "d186" = 1
  dimension "d187" = 1
  dimension "d188" = 1
  constraint parallel L10 L12
  measures "d184" distance of L0.start L10.start
  measures "d185" distance of L4.end L11.start
  measures "d186" distance of L1.end L17.end
  measures "d187" distance of L0.end L15.end
  measures "d188" distance of L13.end L18.end
extrude "Extrude26" cut sketch "Sketch19" against normal blind 2.5 contours L10 L11 L12 L13 L14 L15 L16 L17 L18 L19 bodies 1
extrude "Extrude27" cut 1 faces at (-26.625, -16.9053, 14.3333) along direction (0.503756, -0.863846, 0) blind 0.1 on bodies 1 bodies 1
sketch "Sketch20" plane through (0, 0, 5.5) normal (0, 0, 1) x (-1, 0, 0)
  circle A0 centre (112.0855, -15.5153) radius 2.6
  circle A1 centre (56.1308, -15.5141) radius 2.6
  circle A2 centre (108.184, 14.5373) radius 2.6
  circle A3 centre (84.1085, 23.5123) radius 4.125
  line L0 (93.1085, -17.8627) -> (93.1085, -26.3627)
  line L1 (93.1085, -26.3627) -> (75.1085, -26.3627)
  line L2 (75.1085, -26.3627) -> (75.1085, -17.8627)
  line L3 (75.1085, -17.8627) -> (93.1085, -17.8627)
  arc A4 (46.0033, 0.6373) -> (65.0559, -32.3627) centre (84.1085, 0.6373) ccw
  line L4 (65.0559, -32.3627) -> (103.161, -32.3627)
  arc A5 (103.161, -32.3627) -> (122.2136, 0.6373) centre (84.1085, 0.6373) ccw
  line L5 (122.2136, 0.6373) -> (103.161, 33.6373)
  line L6 (103.161, 33.6373) -> (65.0559, 33.6373)
  line L7 (65.0559, 33.6373) -> (46.0033, 0.6373)
  line L8 (65.0559, 33.6373) -> (68.52, 31.6373)
  line L9 (46.0033, 0.6373) -> (49.4674, -1.3627)
  line L10 (68.52, 31.6373) -> (49.4674, -1.3627)
  line L11 (103.161, 33.6373) -> (103.161, 29.6373)
  line L12 (65.0559, 33.6373) -> (65.0559, 29.6373)
  line L13 (103.161, 29.6373) -> (65.0559, 29.6373)
  line L14 (91.1887, 29.6373) -> (110.9547, -4.5984)
  line L15 (110.9547, -4.5984) -> (93.1085, -22.1127)
  line L16 (75.1085, -22.1127) -> (49.4674, -1.3627)
  dimension "d193" = 4
  dimension "d194" = 4
  dimension "d195" = 4
  dimension "d196" = 4
  constraint coincident L6.end L7.start
  constraint perpendicular L7 L8
  constraint coincident A4.start L7.end
  constraint perpendicular L7 L9
  constraint coincident L5.end L6.start
  constraint perpendicular L6 L11
  constraint perpendicular L6 L12
  constraint coincident L13 L14.start
  constraint parallel L5 L14
  constraint midpoint L0 L15.end
  constraint midpoint L2 L16.start
  measures "d193" distance of L6.end L8.end
  measures "d194" distance of A4.start L9.end
  measures "d195" distance of L5.end L11.end
  measures "d196" distance of L6.end L12.end
extrude "Extrude28" cut sketch "Sketch20" against normal blind 2.5 contours L0 L2 L3 L10 L13 L14 L15 L16 bodies 2
move_body "Move28" bodies 4 to x (0.999657, 0.026177, 0) y (-0.026177, 0.999657, 0) z (0, 0, 1) at (162.7037, 7.0865, 0)
move_body "Move29" bodies 4 to x (1, 0, 0) y (0, 1, 0) z (0, 0, 1) at (0.2906, -0.2078, 0)
move_body "Move30" bodies 4 to x (1, 0, 0) y (0, 1, 0) z (0, 0, 1) at (0, 0, 2)
move_body "Move31" bodies 4 to x (1, 0, 0) y (0, 1, 0) z (0, 0, 1) at (0, 0, -1)
move_body "Move32" bodies 4 to x (1, 0, 0) y (0, 1, 0) z (0, 0, 1) at (0, 0, 0.5)
move_body "Move33" bodies 2 to x (1, 0, 0) y (0, 1, 0) z (0, 0, 1) at (83.417, 1.3029, 0)
move_body "Move34" bodies 6 to x (1, 0, 0) y (0, 1, 0) z (0, 0, 1) at (163.5847, 1.7889, 0)
move_body "Move35" bodies 5 to x (1, 0, 0) y (0, 1, 0) z (0, 0, 1) at (164.0677, 2.0658, 0)
move_body "Move36" bodies 2 to x (1, 0, 0) y (0, 1, 0) z (0, 0, 1) at (-79.1671, -3.9985, 0)
move_body "Move37" bodies 3 to x (1, 0, 0) y (0, 1, 0) z (0, 0, 1) at (163.8283, 3.3526, 0)
move_body "Move38" bodies 6 5 4 3 to x (1, 0, 0) y (0, 1, 0) z (0, 0, 1) at (89.5021, 1.5068, 0)
